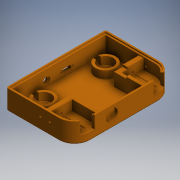
# Autodesk Inventor part: P1794_001
Saved by Autodesk Inventor 2019 (Build 230136000, 136)
## iProperties
Created: 2019-04-29
Part Number: P1794_001
Material: PLA
Document SubType Name: Modeling
Designer: Joan.MAILLARD
Density: 1.25 g/cm^3
Appearance: Orange
Project: P1704 Manette
Description: Bas manette
Author: Joan.MAILLARD
Title: P1704_001_basManette
Autodesk Inventor part; units mm, degrees
ref_plane "YZ Plane" through (0, 0, 0) normal (1, 0, 0) x (0, 1, 0)
ref_plane "XZ Plane" through (0, 0, 0) normal (0, 1, 0) x (-1, 0, 0)
ref_plane "XY Plane" through (0, 0, 0) normal (0, 0, 1) x (1, 0, 0)
sketch "Esquisse1" plane through (0, 0, 0) normal (0, 1, 0) x (-1, 0, 0)
  line L0 (55, 80) -> (55, -80)
  line L1 (-55, -80) -> (-55, 80)
  line L2 (-55, 80) -> (55, -80) construction
  line L3 (55, 80) -> (-55, -80) construction
  line L4 (0, 0) -> (-55, 0) construction
  arc A0 (-55, -55) -> (-30, -80) centre (-30, -55) ccw
  line L5 (-30, -80) -> (55, -80)
  line L6 (-30, -80) -> (-30, -55) construction
  line L7 (55, 80) -> (-30, 80)
  arc A1 (-30, 80) -> (-55, 55) centre (-30, 55) ccw
  line L8 (-30, 55) -> (-30, 80) construction
  dimension "d0" = 160
  dimension "d1" = 110
  dimension "d126" = 25
  dimension "d127" = 25
  constraints: 18 end point, 4 point on circle, 3 horizontal, 3 midpoint, 2 centre point, 2 parallel, 2 point on line, 2 tangent, 2 vertical, 1 perpendicular
  measures "d0" distance of L0.start L0.end
  measures "d1" distance of L0.end L1.start
  measures "d126" distance of L5.start L6.end
  measures "d127" distance of L8.start L7.end
extrude "Extrusion1" add sketch "Esquisse1" along normal blind 32.5
sketch "Esquisse2" plane through (0, 32.5, 0) normal (0, 1, 0) x (1, 0, 0)
  line L0 (-50, 75) -> (-50, -75)
  line L1 (-55, 80) -> (-55, -80) projected
  line L2 (30, 80) -> (-55, 80) projected
  line L3 (-50, -75) -> (30, -75)
  line L4 (30, -75) -> (30, -80) construction
  line L5 (-55, -80) -> (30, -80) construction
  line L6 (-50, 75) -> (30, 75)
  line L7 (30, 75) -> (30, 80) construction
  arc A0 (50, 55) -> (30, 75) centre (30, 55) ccw
  line L8 (30, 75) -> (30, 55) construction
  arc A1 (55, 55) -> (30, 80) centre (30, 55) ccw construction
  line L9 (50, 55) -> (50, -55)
  line L10 (55, 55) -> (50, 55) construction
  line L11 (50, -55) -> (55, -55) construction
  arc A2 (30, -75) -> (50, -55) centre (30, -55) ccw
  line L12 (55, -55) -> (55, 55) construction
  point P0 (0, 0)
  dimension "d67" = 5
  dimension "d131" = 5
  constraints: 18 end point, 4 horizontal, 4 point on circle, 3 vertical, 2 centre point, 2 tangent, 1 coincident, 1 concentric, 1 parallel, 1 perpendicular
  measures "d67" distance between parallel lines of L1 L0
  measures "d131" distance between parallel lines of L12 L9
extrude "Extrusion2" cut sketch "Esquisse2" against normal blind 27.5
sketch "Esquisse6" plane through (0, 5, 0) normal (0, 1, 0) x (1, 0, 0)
  line L0 (50, 40) -> (11.25, 40)
  line L1 (11.25, 40) -> (11.25, 35)
  line L2 (11.25, 35) -> (50, 35)
  line L3 (50, 35) -> (50, 40)
  line L4 (11.25, 35) -> (3.75, 35)
  line L5 (3.75, 35) -> (3.75, 75)
  line L6 (3.75, 75) -> (11.25, 75)
  line L7 (11.25, 75) -> (11.25, 35)
  line L8 (11.25, -75) -> (3.75, -75)
  line L9 (3.75, -75) -> (3.75, -35)
  line L10 (3.75, -35) -> (11.25, -35)
  line L11 (11.25, -35) -> (11.25, -75)
  line L12 (50, -35) -> (11.25, -35)
  line L13 (11.25, -35) -> (11.25, -40)
  line L14 (11.25, -40) -> (50, -40)
  line L15 (50, -40) -> (50, -35)
  line L16 (11.25, -75) -> (80.7095, -75) construction
  line L17 (50, -40) -> (50, -93.5027) construction
  line L18 (30, -75) -> (-50, -75) construction
  line L19 (50, 55) -> (50, -55) construction
  line L20 (-50, 75) -> (30, 75) construction
  point P0 (0, 0)
  point P1 (7.5, -35)
  dimension "d44" = 5
  dimension "d45" = 7.5
  dimension "d48" = 5
  dimension "d50" = 7.5
  dimension "d132" = 35
  dimension "d133" = 38.75
  dimension "d134" = 38.75
  dimension "d135" = 35
  constraints: 36 end point, 8 parallel, 5 horizontal, 5 point on line, 4 perpendicular, 1 midpoint, 1 vertical
  measures "d44" distance between parallel lines of L2 L0
  measures "d45" distance between parallel lines of L5 L7
  measures "d48" distance between parallel lines of L14 L12
  measures "d50" distance between parallel lines of L11 L9
  measures "d132" distance between parallel lines of L14 L16
  measures "d133" distance between parallel lines of L11 L17
  measures "d134" distance of L0.start L0.end
  measures "d135" distance between parallel lines of L20 L0
extrude "Extrusion4" add sketch "Esquisse6" along normal blind 24
sketch "Esquisse11" plane through (55, 0, 55) normal (1, 0, 0) x (0, 0, -1)
  line L0 (-12.5, 32.5) -> (7.5, 32.5)
  line L1 (7.5, 32.5) -> (7.5, 12.5)
  line L2 (7.5, 12.5) -> (-12.5, 12.5)
  line L3 (-12.5, 12.5) -> (-12.5, 32.5)
  line L4 (122.5, 32.5) -> (102.5, 32.5)
  line L5 (102.5, 32.5) -> (102.5, 12.5)
  line L6 (102.5, 12.5) -> (122.5, 12.5)
  line L7 (122.5, 12.5) -> (122.5, 32.5)
  line L8 (0, 0) -> (110, 0) projected
  line L9 (0, 32.5) -> (110, 32.5) projected
  line L10 (135, 0) -> (110, 0) projected
  line L11 (135, 32.5) -> (110, 32.5) projected
  line L12 (-25, 0) -> (-25, 32.5) projected
  line L13 (135, 0) -> (135, 32.5) projected
  line L14 (71.6904, 12.5) -> (52.7334, 12.5) construction
  dimension "d138" = 20
  dimension "d139" = 20
  dimension "d140" = 12.5
  dimension "d141" = 12.5
  dimension "d154" = 12.5
  constraints: 18 end point, 4 parallel, 3 collinear, 3 horizontal, 2 perpendicular, 1 coincident, 1 midpoint, 1 point on line
  measures "d138" distance between parallel lines of L3 L1
  measures "d139" distance between parallel lines of L7 L5
  measures "d140" distance between parallel lines of L12 L3
  measures "d141" distance between parallel lines of L13 L7
  measures "d154" distance between parallel lines of L14 L10
extrude "Extrusion6" cut sketch "Esquisse11" against normal blind 20
sketch "Esquisse16" plane through (11.25, 5, 75) normal (1, 0, 0) x (0, 0, -1)
  line L0 (17.5, 12.5) -> (7.5, 12.5) construction
  line L1 (17.5, 12.5) -> (27.5, 12.5) construction
  line L2 (130, 0) -> (122.5, 0) construction
  line L3 (7.5, 7.5) -> (7.5, 27.5) projected
  line L4 (27.5, 27.5) -> (27.5, 7.5) projected
  line L5 (7.5, 6) -> (20, 6) projected
  line L6 (27.5, 7.5) -> (20, 7.5) projected
  point P0 (75, -5)
  point P1 (130, 6)
  point P2 (122.5, 6)
  point P3 (27.5, 6)
  point P4 (27.5, -5)
  dimension "d174" = 5
  constraints: 4 end point, 3 point on line, 1 collinear, 1 horizontal, 1 other
  measures "d174" distance between parallel lines of L1 L6
hole "Perçage6" at (11.25, 17.5, 57.5) direction (-1, 0, 0) diameter 3.4 depth 10
sketch "Esquisse17" plane through (11.25, 5, -40) normal (1, 0, 0) x (0, 0, -1)
  line L0 (27.5, 27.5) -> (27.5, 7.5) projected
  line L1 (7.5, 7.5) -> (7.5, 27.5) projected
  line L2 (5.8848, 12.5) -> (-4.3187, 12.5) construction
  line L3 (15, 7.5) -> (15, 7.5) projected
  line L4 (17.5, 12.5) -> (7.5, 12.5) construction
  line L5 (17.5, 12.5) -> (27.5, 12.5) construction
  point P0 (-40, -5)
  point P1 (7.5, 6)
  point P2 (-87.5, 6)
  point P3 (27.5, -5)
  point P4 (7.5, -5)
  dimension "d155" = 5
  constraints: 6 end point, 3 point on line, 2 perpendicular, 1 collinear, 1 horizontal, 1 horizontal alignment
hole "Perçage7" at (11.25, 17.5, -57.5) direction (-1, 0, 0) diameter 3.4 depth 10
sketch "Esquisse20" plane through (0, 32.5, 0) normal (0, 1, 0) x (1, 0, 0)
  line L0 (-52.5, 77.5) -> (-52.5, -77.5)
  line L1 (-52.5, -77.5) -> (30, -77.5)
  arc A0 (30, -77.5) -> (52.5, -55) centre (30, -55) ccw
  line L2 (52.5, -55) -> (52.5, 55)
  arc A1 (52.5, 55) -> (30, 77.5) centre (30, 55) ccw
  line L3 (-52.5, 77.5) -> (30, 77.5)
  line L4 (30, 80) -> (30, 75) construction
  arc A2 (45.6125, 67.5) -> (30, 75) centre (30, 55) ccw construction
  line L5 (30, -80) -> (30, -75) construction
  arc A3 (30, -80) -> (51.6506, -67.5) centre (30, -55) ccw construction
  arc A4 (51.6506, 67.5) -> (30, 80) centre (30, 55) ccw construction
  line L6 (-50, 0) -> (-55, 0) construction
  line L7 (-55, 0) -> (-50, 0) construction
  line L8 (-50, -75) -> (-50, 75) construction
  line L9 (-55, 80) -> (-55, -80) construction
  line L10 (30, 75) -> (-50, 75)
  line L11 (-50, -75) -> (30, -75)
  arc A5 (50, 55) -> (30, 75) centre (30, 55) ccw
  arc A6 (30, -75) -> (50, -55) centre (30, -55) ccw
  line L12 (50, -55) -> (50, 55)
  point P0 (0, 0)
  point P1 (-52.5, 0)
  constraints: 22 end point, 12 point on circle, 6 midpoint, 5 horizontal, 5 tangent, 4 centre point, 4 vertical, 3 concentric, 2 coincident, 2 equal radius, 2 parallel, 1 collinear
extrude "Extrusion12" cut sketch "Esquisse20" against normal blind 2
sketch "Esquisse22" plane through (0, 5, 0) normal (0, 1, 0) x (1, 0, 0)
  line L0 (11.25, -75) -> (11.25, -40) projected
  line L1 (11.25, -40) -> (11.25, -75) projected
  line L2 (30, -75) -> (11.25, -75) projected
  arc A0 (30, -75) -> (50, -55) centre (30, -55) ccw projected
  line L3 (50, -40) -> (50, -55) projected
  line L4 (50, -40) -> (11.25, -40) projected
  line L5 (11.25, 75) -> (11.25, 40) projected
  line L6 (11.25, 40) -> (50, 40) projected
  line L7 (50, 55) -> (50, 40) projected
  arc A1 (50, 55) -> (30, 75) centre (30, 55) ccw projected
  line L8 (11.25, 75) -> (30, 75) projected
  point P0 (0, 0)
extrude "Extrusion14" add sketch "Esquisse22" along normal blind 7.5
sketch "Esquisse24" plane through (55, 12.5, 55) normal (0, 1, 0) x (1, 0, 0)
  line L0 (-9.3875, -7.5596) -> (-9.3875, 12.2233) construction
  line L1 (-43.75, -7.1) -> (-9.3875, -7.1)
  line L2 (-9.3875, -7.1) -> (-9.3875, -6.1)
  line L3 (-9.3875, -6.1) -> (-43.75, -6.1)
  line L4 (-43.75, -6.1) -> (-43.75, -7.1)
  line L5 (-43.75, 1.1) -> (-9.3875, 1.1)
  line L6 (-9.3875, 1.1) -> (-9.3875, 2.1)
  line L7 (-9.3875, 2.1) -> (-43.75, 2.1)
  line L8 (-43.75, 2.1) -> (-43.75, 1.1)
  line L9 (-43.75, -20) -> (-43.75, 15) construction
  line L10 (-43.75, 15) -> (-5, 15) projected
  line L11 (-43.75, 107.9) -> (-9.3875, 107.9)
  line L12 (-9.3875, 107.9) -> (-9.3875, 108.9)
  line L13 (-9.3875, 108.9) -> (-43.75, 108.9)
  line L14 (-43.75, 108.9) -> (-43.75, 107.9)
  line L15 (-43.75, 116.1) -> (-9.3875, 116.1)
  line L16 (-9.3875, 116.1) -> (-9.3875, 117.1)
  line L17 (-9.3875, 117.1) -> (-43.75, 117.1)
  line L18 (-43.75, 117.1) -> (-43.75, 116.1)
  line L19 (-5, 95) -> (-43.75, 95) projected
  line L20 (-43.75, 95) -> (-43.75, 130) projected
  point P0 (-9.3875, -12.5)
  point P1 (-43.75, 1.6)
  point P2 (-43.75, -6.6)
  point P3 (-9.3875, 1.6)
  point P4 (-9.3875, -6.6)
  point P5 (-9.3875, 108.4)
  point P6 (-9.3875, 116.6)
  point P7 (-43.75, 108.4)
  dimension "d160" = 1
  dimension "d161" = 1
  dimension "d162" = 7.2
  dimension "d163" = 12.9
  dimension "d164" = 1
  dimension "d165" = 1
  dimension "d166" = 7.2
  dimension "d167" = 12.9
  constraints: 34 end point, 9 point on line, 8 parallel, 7 midpoint, 4 horizontal, 4 perpendicular, 1 vertical
  measures "d160" distance of L1.end L2.end
  measures "d161" distance of L5.end L6.end
  measures "d162" distance between parallel lines of L3 L5
  measures "d163" distance between parallel lines of L10 L7
  measures "d164" distance of L15.end L16.end
  measures "d165" distance of L11.end L12.end
  measures "d166" distance between parallel lines of L15 L13
  measures "d167" distance between parallel lines of L11 L19
extrude "Extrusion15" add sketch "Esquisse24" along normal blind 0.9
sketch "Esquisse25" plane through (0, 29, 0) normal (0, 1, 0) x (1, 0, 0)
  line L0 (3.75, 35) -> (23.25, 35)
  line L1 (23.25, 35) -> (23.25, 49)
  line L2 (23.25, 49) -> (3.75, 49)
  line L3 (3.75, 49) -> (3.75, 35)
  line L4 (3.75, 75) -> (3.75, 35) construction
  line L5 (3.75, 35) -> (50, 35) construction
  point P0 (0, 0)
  dimension "d170" = 14
  dimension "d171" = 19.5
  constraints: 8 end point, 2 collinear, 2 parallel, 1 horizontal, 1 perpendicular
  measures "d170" distance of L0.end L1.end
  measures "d171" distance between parallel lines of L3 L1
extrude "Extrusion16" cut sketch "Esquisse25" against normal blind 3
sketch "Esquisse26" plane through (0, 0, 0) normal (0, -1, 0) x (1, 0, 0)
  line L0 (50, 47.5) -> (50, -47.5) projected
  line L1 (30, -75) -> (-50, -75) projected
  point P0 (0, 0)
  point P1 (43.904, 1.2)
  dimension "d196" = 6.096
  dimension "d197" = 76.2
  measures "d196" distance from line of L0 point (43.904, 1.2)
  measures "d197" distance from line of point (43.904, 1.2) L1
hole "Perçage8" at (43.904, 0, 1.2) direction (0, 1, 0) diameter 3.4 end through all countersink diameter 6.3 countersink angle 90
sketch "Esquisse27" plane through (0, 0, 0) normal (0, -1, 0) x (1, 0, 0)
  line L0 (-50, -75) -> (3.75, -75) projected
  line L1 (50, -35) -> (50, 35) projected
  point P0 (0, 0)
  point P1 (-43.98, 69.78)
  dimension "d198" = 144.78
  dimension "d199" = 93.98
  measures "d198" distance from line of L0 point (-43.98, 69.78)
  measures "d199" distance from line of L1 point (-43.98, 69.78)
hole "Perçage9" at (-43.98, 0, 69.78) direction (0, 1, 0) diameter 3.4 end through all countersink diameter 6.3 countersink angle 90
sketch "Esquisse28" plane through (0, 0, 0) normal (0, -1, 0) x (1, 0, 0)
  line L0 (-50, -75) -> (3.75, -75) projected
  line L1 (-50, 75) -> (-50, -75) projected
  line L2 (55, 55) -> (55, -55) projected
  line L3 (50, 47.5) -> (50, -47.5) projected
  point P0 (0, 0)
  point P1 (-44.488, -68.904)
  dimension "d200" = 6.096
  dimension "d203" = 94.488
  measures "d200" distance from line of L0 point (-44.488, -68.904)
  measures "d203" distance from line of L3 point (-44.488, -68.904)
hole "Perçage10" at (-44.488, 0, -68.904) direction (0, 1, 0) diameter 3.4 end through all countersink diameter 6.3 countersink angle 90
sketch "Esquisse29" plane through (-55, 0, -80) normal (-1, 0, 0) x (0, 0, 1)
  line L0 (0, 0) -> (0, 32.5) projected
  line L1 (0, 0) -> (160, 0) projected
  point P0 (80, 0)
  point P1 (58, 14)
  dimension "d211" = 58
  dimension "d212" = 14
  measures "d211" distance from line of L0 point (58, 14)
  measures "d212" distance from line of L1 point (58, 14)
hole "Perçage11" at (-55, 14, -22) direction (1, 0, 0) diameter 2.9 depth 5 tip angle 118
pattern_linear "Réseau rectangulaire1" count 2 spacing 19 along (0, 0, 1) of "Perçage11"
sketch "Esquisse30" plane through (-55, 0, -80) normal (-1, 0, 0) x (0, 0, 1)
  line L0 (61, 11) -> (74, 11)
  line L1 (74, 11) -> (74, 17)
  line L2 (74, 17) -> (61, 17)
  line L3 (61, 17) -> (61, 11)
  circle A0 centre (77, 14) radius 1.45 projected
  circle A1 centre (58, 14) radius 1.45 projected
  line L4 (42.6122, -10.7376) -> (49.1431, -10.7376)
  line L5 (61, 11) -> (74, 17) construction
  line L6 (74, 11) -> (61, 17) construction
  line L7 (67.5, 14) -> (58, 14) construction
  line L8 (67.5, 14) -> (77, 14) construction
  point P0 (80, 0)
  dimension "d216" = 13
  dimension "d217" = 6
  constraints: 18 end point, 4 horizontal, 2 parallel, 1 collinear, 1 midpoint, 1 perpendicular
  measures "d216" distance of L0.start L0.end
  measures "d217" distance of L0.end L1.end
extrude "Extrusion17" cut sketch "Esquisse30" against normal blind 10 contours L3 L2 L1 L0
sketch "Esquisse32" plane through (-50, 5, 75) normal (1, 0, 0) x (0, 0, -1)
  line L0 (155, -5) -> (-5, -5) projected
  line L1 (-5, -5) -> (-5, 27.5) projected
  point P0 (75, -5)
  point P1 (55, 9)
  dimension "d235" = 14
  dimension "d236" = 60
  measures "d235" distance from line of L0 point (55, 9)
  measures "d236" distance from line of L1 point (55, 9)
hole "Perçage13" at (-50, 14, 20) direction (-1, 0, 0) diameter 7.2 end through all counterbore diameter 11 counterbore depth 2
sketch "Esquisse33" plane through (55, 0, 55) normal (1, 0, 0) x (0, 0, -1)
  arc A0 (37.7423, 9.55) -> (32.2577, 9.55) centre (35, 18.75) ccw
  line L0 (135, 0) -> (135, 32.5) projected
  line L1 (-25, 0) -> (-25, 32.5) projected
  line L2 (35, 18.75) -> (35, 5)
  line L3 (35, 32.5) -> (35, 18.75)
  line L4 (122.204, 5) -> (125.604, 5) projected
  line L5 (-16.48, 5) -> (-13.08, 5) projected
  line L6 (52.1, 5) -> (55.5, 5) construction
  line L7 (-20, 5) -> (20, 5) construction
  line L8 (90, 5) -> (20, 5) construction
  line L9 (90, 5) -> (130, 5) construction
  line L10 (-20, 5) -> (130, 5) construction
  line L11 (7.5, 32.5) -> (102.5, 32.5) projected
  line L12 (37.7423, 9.55) -> (32.2577, 9.55)
  point P0 (55, 0)
  dimension "d239" = 9.6
  dimension "d242" = 100
  dimension "d277" = 9.2
  constraints: 6 end point, 2 point on circle, 2 point on line, 2 vertical, 1 centre point, 1 coincident, 1 collinear, 1 horizontal
  measures "d239" radius of A0
  measures "d242" distance from line of L0 A0.centre
  measures "d277" distance from line of L12 A0.centre
extrude "Extrusion18" cut sketch "Esquisse33" against normal up to next
sketch "Esquisse34" plane through (0, 5, 0) normal (0, 1, 0) x (1, 0, 0)
  arc A0 (-36.5785, -54) -> (-36.5785, -46) centre (-25, -50) ccw
  arc A1 (-40.75, -54) -> (-40.75, -46) centre (-25, -50) ccw
  line L0 (-40.75, -46) -> (-36.5785, -46)
  line L1 (-40.75, -54) -> (-36.5785, -54)
  line L2 (-36.5785, -36.3891) -> (-36.5785, -60.826) construction
  arc A2 (-36.5785, 46) -> (-36.5785, 54) centre (-25, 50) ccw
  arc A3 (-40.75, 46) -> (-40.75, 54) centre (-25, 50) ccw
  line L3 (-40.75, 54) -> (-36.5785, 54)
  line L4 (-40.75, 46) -> (-36.5785, 46)
  line L5 (-36.5785, 54.2054) -> (-36.5785, 29.7686) construction
  line L6 (-25, 118.9857) -> (-25, 88.2412) construction
  line L7 (-55, 80) -> (-55, -80) projected
  line L8 (-77, 0) -> (77, 0) construction
  line L9 (-25, 50) -> (-25, 0) construction
  line L10 (-25, 0) -> (-25, -50) construction
  point P0 (0, 0)
  dimension "d243" = 4
  dimension "d244" = 12.25
  dimension "d245" = 8
  dimension "d246" = 4
  dimension "d247" = 12.25
  dimension "d248" = 8
  dimension "d249" = 30
  dimension "d250" = 50
  constraints: 18 end point, 8 point on circle, 7 point on line, 4 centre point, 4 horizontal, 4 vertical, 2 concentric, 1 collinear, 1 perpendicular
  measures "d243" radial gap between concentric circles of A1 A0
  measures "d244" radius of A0
  measures "d245" distance between parallel lines of L0 L1
  measures "d246" radial gap between concentric circles of A3 A2
  measures "d247" radius of A2
  measures "d248" distance between parallel lines of L3 L4
  measures "d249" distance between parallel lines of L7 L6
  measures "d250" distance of L9.end L10.end
extrude "Extrusion19" add sketch "Esquisse34" along normal blind 12.5
sketch "Esquisse35" plane through (30, 0, -80) normal (0, 0, -1) x (-1, 0, 0)
  line L0 (0, 0) -> (85, 0) projected
  line L1 (85, 0) -> (85, 32.5) projected
  point P0 (30, 0)
  point P1 (15, 19)
  dimension "d263" = 19
  dimension "d264" = 70
  measures "d263" distance from line of L0 point (15, 19)
  measures "d264" distance from line of L1 point (15, 19)
hole "Perçage14" at (15, 19, -80) direction (0, 0, 1) diameter 3.4 depth 5 tip angle 118
pattern_linear "Réseau rectangulaire2" count 2 spacing 15 along (-1, 0, 0) of "Perçage14"
sketch "Esquisse36" plane through (-55, 0, 80) normal (0, 0, 1) x (1, 0, 0)
  line L0 (0, 0) -> (85, 0) projected
  line L1 (0, 0) -> (0, 32.5) projected
  point P0 (55, 0)
  point P1 (70, 19)
  dimension "d275" = 19
  dimension "d276" = 70
  measures "d275" distance from line of L0 point (70, 19)
  measures "d276" distance from line of L1 point (70, 19)
hole "Perçage15" at (15, 19, 80) direction (0, 0, -1) diameter 3.4 depth 5 tip angle 118
pattern_linear "Réseau rectangulaire3" count 2 spacing 15 along (-1, 0, 0) of "Perçage15"
fillet "Congé3" radius 3 8 edges at (-55, 16.25, -80) (-55, 16.25, 80) (47.6777, 0, 72.6777) (55, 0, 0) (47.6777, 0, -72.6777) (-12.5, 0, -80) (-12.5, 0, 80) (-55, 0, 0)
equation "\"d67\" = d66"
equation "\"d131\" = d67"
equation "\"d45\" = 1.5 * d44"
equation "\"d48\" = d44"
equation "\"d50\" = d45"
equation "\"d134\" = d133"
equation "\"d135\" = d132"
equation "\"d139\" = d138"
equation "\"d141\" = d140"
equation "\"d66\" = 5"
